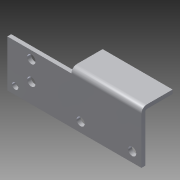
# Autodesk Inventor part: endstop
Saved by Autodesk Inventor 2013 (Build 170138000, 138)
## iProperties
Created: 2013-01-24
Part Number: endstop
Material: Aluminum 6061
Document SubType Name: Sheet Metal
Designer: Arpan
Density: 2.71 g/cm^3
Sheet Metal Rule: Default
Mass: 44.7583 g
Surface Area: 117.075 cm^2
Volume: 16.516 cm^3
Flat Pattern Width: 10.9144 cm
Flat Pattern Length: 6.32443 cm
Flat Pattern Area: 69.0272 cm^2
Sheet Metal Width: 4.297 in
Sheet Metal Length: 2.490 in
Sheet Metal Area: 10.699 in^2
Author: Arpan
Autodesk Inventor part; units mm, degrees
ref_plane "YZ Plane" through (0, 0, 0) normal (1, 0, 0) x (0, 1, 0)
ref_plane "XZ Plane" through (0, 0, 0) normal (0, 1, 0) x (-1, 0, 0)
ref_plane "XY Plane" through (0, 0, 0) normal (0, 0, 1) x (1, 0, 0)
sketch "Sketch1" plane through (0, 0, 0) normal (0, 0, 1) x (1, 0, 0)
  line L0 (0, 0) -> (-109.1438, 0)
  line L1 (-109.1438, 0) -> (-109.1438, 38.1)
  line L2 (-109.1438, 38.1) -> (0, 38.1)
  line L3 (0, 38.1) -> (0, 0)
  line L4 (0, 38.1) -> (-7.493, 38.1)
  line L5 (-7.493, 38.1) -> (-7.493, 8.1026)
  line L6 (-109.1438, 38.1) -> (-101.6508, 38.1)
  line L7 (-101.6508, 38.1) -> (-101.6508, 8.1026)
  dimension "d1" = 109.1438
  dimension "d2" = 38.1
  dimension "d3" = 7.493
  dimension "d4" = 29.9974
  dimension "d5" = 7.493
  measures "d1" distance of L0.start L0.end
  measures "d2" distance of L0.end L1.end
  measures "d3" distance of L2.end L4.end
  measures "d4" distance of L4.end L5.end
  measures "d5" distance of L1.end L6.end
extrude "Plate1" add sketch "Sketch1" along normal blind 3.175
sketch "Sketch2" plane through (0, 39.37, -1.27) normal (0, 1, 0) x (-1, 0, 0)
  line L0 (109.1438, 0) -> (0, 0)
  line L1 (0, 0) -> (0, -20.955)
  line L2 (0, -20.955) -> (109.1438, -20.955)
  line L3 (109.1438, -20.955) -> (109.1438, 0)
  constraints: 6 end point, 1 horizontal, 1 perpendicular, 1 vertical
edge flange "Flange1" height 25.4 angle 90 thickness 3.175 bend radius 1.27 thickness toward (0, 1, 0) relief straight relief width 3.175 relief depth 1.5875 corner gap 3.175 corner form 0 edges at (-105.3973, 38.1, 0) (-54.5719, 38.1, 0) (-3.7465, 38.1, 0) wall of the first edge with corners at (-109.1438, 39.37, -1.27) (0, 39.37, -1.27) (0, 39.37, -22.225) (-109.1438, 39.37, -22.225)
bend "Bend1"
corner "Corner1"
sketch "Sketch8" plane through (0, 0, 3.175) normal (0, 0, 1) x (1, 0, 0)
  circle A0 centre (-7.5, 7.9) radius 3.3 projected
  circle A1 centre (-49.5, 7.9) radius 3.3 projected
extrude "Cut1" cut sketch "Sketch8" against normal blind 3.175
sketch "Sketch10" plane through (0, 0, 3.175) normal (0, 0, 1) x (1, 0, 0)
  line L0 (-109.1438, 38.1) -> (0, 38.1) projected
  line L1 (-109.1438, 0) -> (-109.1438, 38.1) projected
  line L2 (-109.1438, 38.1) -> (-109.1438, 88.9)
  line L3 (-109.1438, 88.9) -> (-56.9976, 88.9)
  line L4 (-56.9976, 88.9) -> (-56.9976, 38.1)
  dimension "d21" = 50.8
  dimension "d22" = 52.1462
  constraints: 6 end point, 2 perpendicular, 1 collinear, 1 point on line
  measures "d21" distance of L0.start L2.end
  measures "d22" distance of L2.end L3.end
extrude "Extrusion1" cut sketch "Sketch10" against normal blind 25.4
sketch "Sketch15" plane through (0, 0, 3.175) normal (0, 0, 1) x (1, 0, 0)
  line L0 (0, 0) -> (-109.1438, 0) projected
  line L1 (-109.1438, 0) -> (-102.7938, 0)
  line L2 (-102.7938, 0) -> (-102.7938, 6.35)
  circle A0 centre (-102.7938, 6.35) radius 2.54
  dimension "d31" = 6.35
  dimension "d32" = 6.35
  dimension "d33" = 5.08
  constraints: 4 end point, 1 centre point, 1 coincident, 1 perpendicular, 1 point on line
  measures "d31" distance of L0.end L1.end
  measures "d32" distance of L1.end L2.end
  measures "d33" diameter of A0
extrude "Cut4" cut sketch "Sketch15" against normal blind 3.175
sketch "Sketch16" plane through (0, 0, 3.175) normal (0, 0, 1) x (1, 0, 0)
  circle A0 centre (-90.6026, 15.875) radius 3.3782
  circle A1 centre (-90.6026, 31.75) radius 3.3782
  constraints: 2 centre point, 4 other
extrude "Cut5" cut sketch "Sketch16" against normal blind 3.175
equation "\"d19\" = Thickness"
equation "\"d34\" = Thickness"
equation "\"d36\" = Thickness"
equation "\"d9\" = BendReliefWidth"
equation "\"d10\" = BendReliefDepth"
equation "\"d11\" = MinimumRemnant"
equation "\"d12\" = BendRadius"
equation "\"d16\" = CornerReliefSize"
equation "\"d17\" = GapSize"
equation "\"d18\" = JacobiRadiusSize"
equation "\"BendRadius\" = Thickness"
equation "\"BendReliefWidth\" = Thickness"
equation "\"BendReliefDepth\" = 0.5 * Thickness"
equation "\"CornerReliefSize\" = 4 * Thickness"
equation "\"MinimumRemnant\" = 2 * Thickness"
equation "\"TransitionRadius\" = BendRadius"
equation "\"JacobiRadiusSize\" = BendRadius"
equation "\"GapSize\" = Thickness"
equation "\"d8\" = BendRadius"
equation "\"Thickness\" = 3.175"
body "Solid1"
